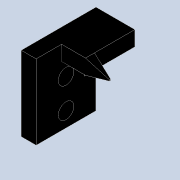
# Autodesk Inventor part: Z Axis Limt Adjustable Trigger
Saved by Autodesk Inventor 2022 (Build 260153000, 153)
## iProperties
Created: 2021-10-25
Part Number: Z Axis Limt Adjustable Trigger
Material: Generic
Document SubType Name: Modeling
Designer: Coy
Density: 1 g/cm^3
Appearance: Anodized - Black
Author: Coy
Autodesk Inventor part; units mm, degrees
ref_plane "YZ Plane" through (0, 0, 0) normal (1, 0, 0) x (0, 1, 0)
ref_plane "XZ Plane" through (0, 0, 0) normal (0, 1, 0) x (-1, 0, 0)
sketch "Sketch1" plane through (0, 0, 0) normal (1, 0, 0) x (0, 1, 0)
  line L0 (0, 0) -> (5, 0)
  line L1 (5, 0) -> (5, -25)
  line L2 (5, -25) -> (0, -25)
  line L3 (0, -25) -> (0, 0)
  line L4 (0, 0) -> (-20, 0)
  line L5 (-20, 0) -> (-20, -20)
  line L6 (-20, -20) -> (0, -20)
  line L7 (0, -20) -> (0, 0)
  line L8 (-20, -10) -> (0, -10) construction
  circle A0 centre (-5, -10) radius 2.6
  circle A1 centre (-15, -10) radius 2.6
  dimension "d0" = 5
  dimension "d1" = 25
  dimension "d2" = 20
  dimension "d3" = 20
  dimension "d4" = 5.2
  dimension "d5" = 5.2
  dimension "d6" = 5
  dimension "d7" = 5
  constraints: 18 end point, 4 parallel, 2 centre point, 2 horizontal, 2 midpoint, 2 perpendicular, 2 point on line
  measures "d0" distance of L1.end L2.end
  measures "d1" distance of L0.end L1.end
  measures "d2" distance of L6.end L5.end
  measures "d3" distance of L5.end L4.end
  measures "d4" diameter of A0
  measures "d5" diameter of A1
  measures "d6" distance from line of L3 A0.centre
  measures "d7" distance from line of L5 A1.centre
extrude "Extrusion1" add sketch "Sketch1" along normal blind 5
sketch "Sketch2" plane through (5, 0, 0) normal (1, 0, 0) x (0, 0, -1)
  line L0 (20, 0) -> (25, 0) projected
  line L1 (25, 5) -> (0, 5) projected
  line L2 (25, 0) -> (0, 0)
  line L3 (0, 0) -> (0, 5)
  line L4 (0, 5) -> (25, 5)
  line L5 (25, 5) -> (25, 0)
  line L6 (0, 0) -> (4, 0)
  line L7 (4, 0) -> (4, -8)
  line L8 (4, -8) -> (0, -8)
  line L9 (0, -8) -> (0, 0)
  line L10 (20, -20) -> (20, 0) projected
  line L11 (20, 0) -> (16, 0)
  line L12 (16, 0) -> (16, -8)
  line L13 (16, -8) -> (20, -8)
  line L14 (20, -8) -> (20, 0)
  line L15 (8.5, 0) -> (8.5, 5)
  point P0 (8.5, 5)
  dimension "d12" = 4
  dimension "d13" = 8
  dimension "d14" = 4
  dimension "d15" = 8
  dimension "d19" = 8.5
  constraints: 26 end point, 6 parallel, 4 perpendicular, 3 horizontal, 2 point on line
  measures "d12" distance of L7.end L8.end
  measures "d13" distance of L6.end L7.end
  measures "d14" distance of L13.end L12.end
  measures "d15" distance of L12.end L11.end
  measures "d19" distance between parallel lines of L3 L15
extrude "Extrusion2" add sketch "Sketch2" along normal blind 8 contours L2 L15 L1 L5 L0 | L10 L13 L12 L2
chamfer "Chamfer1" distance 8 angle 45 1 edges at (13, -8, -18)
sketch "Sketch3" plane through (13, 0, 0) normal (1, 0, 0) x (0, 0, -1)
  line L0 (8.5, 0) -> (8.5, 5) projected
  line L1 (16, 0) -> (8.5, 0) projected
  line L2 (8.5, 5) -> (8.5, 0)
  line L3 (8.5, 0) -> (11.5, 0)
  line L4 (11.5, 0) -> (11.5, 5)
  line L5 (25, 5) -> (0, 5) projected
  line L6 (11.5, 5) -> (8.5, 5)
  point P0 (0, 0)
  dimension "d20" = 3
  constraints: 8 end point, 2 point on line, 1 perpendicular, 1 vertical
  measures "d20" distance of L0.start L3.end
ref_plane "Work Plane1" through (21, 0, 0) normal (1, 0, 0) x (0, 0, -1)
sketch "Sketch4" plane through (21, 0, 0) normal (1, 0, 0) x (0, 0, -1)
  line L0 (8.5, 0) -> (8.5, 5) construction
  line L1 (8.5, 2.5) -> (11.5, 2.5) construction
  line L2 (25, 5) -> (0, 5) construction
  line L3 (8.5, 2.7) -> (8.9, 2.7)
  line L4 (8.9, 2.7) -> (8.9, 2.3)
  line L5 (8.9, 2.3) -> (8.5, 2.3)
  line L6 (8.5, 2.3) -> (8.5, 2.7)
  point P0 (0, 0)
  dimension "d22" = 3
  dimension "d23" = 0.2
  dimension "d24" = 0.2
  dimension "d25" = 0.4
  constraints: 10 end point, 2 parallel, 2 perpendicular, 1 horizontal, 1 midpoint, 1 point on line
  measures "d22" distance of L1.start L1.end
  measures "d23" distance between parallel lines of L1 L3
  measures "d24" distance between parallel lines of L1 L5
  measures "d25" distance between parallel lines of L0 L4
loft "Loft1" add profiles "Sketch3", "Sketch4"
equation "\"d7\" = d6"
equation "\"d24\" = d23"
body "Solid1"
